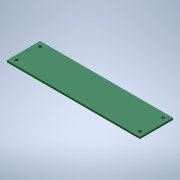
# Autodesk Inventor part: tapa
Saved by Autodesk Inventor 2021 (Build 250183000, 183)
## iProperties
Created: 2021-03-08
Part Number: tapa
Material: Steel, Mild, Welded
Document SubType Name: Modeling
Designer: Usuario
Density: 7.85 g/cm^3
Appearance: Smooth - Dark Sea Green
Author: Usuario
Autodesk Inventor part; units mm, degrees
ref_plane "YZ Plane" through (0, 0, 0) normal (1, 0, 0) x (0, 1, 0)
ref_plane "XZ Plane" through (0, 0, 0) normal (0, 1, 0) x (-1, 0, 0)
ref_plane "XY Plane" through (0, 0, 0) normal (0, 0, 1) x (1, 0, 0)
sketch "Sketch1" plane through (0, 0, 0) normal (0, 1, 0) x (-1, 0, 0)
  line L0 (76, 19) -> (-76, 19)
  line L1 (-76, 19) -> (-76, -19)
  line L2 (-76, -19) -> (76, -19)
  line L3 (76, -19) -> (76, 19)
  line L4 (76, 19) -> (-76, -19) construction
  line L5 (-76, 19) -> (76, -19) construction
  point P0 (0, 0)
  dimension "d0" = 152
  dimension "d1" = 38
  constraints: 12 end point, 2 midpoint, 2 parallel, 1 horizontal, 1 perpendicular
  measures "d0" distance of L2.end L1.end
  measures "d1" distance of L1.end L0.end
extrude "Extrusion1" add sketch "Sketch1" along normal blind 2
sketch "Sketch2" plane through (0, 0, 0) normal (0, -1, 0) x (1, 0, 0)
  line L0 (76, 19) -> (76, -19) projected
  line L1 (-76, 19) -> (76, 19) projected
  line L2 (-76, -19) -> (-76, 19) projected
  line L3 (76, -19) -> (-76, -19) projected
  line L4 (-76, -19) -> (-76, 19) projected
  line L5 (-76, 19) -> (76, 19) projected
  line L6 (-76, -19) -> (76, -19)
  line L7 (76, -19) -> (76, 19)
  line L8 (76, 19) -> (-76, 19)
  line L9 (-76, 19) -> (-76, -19)
  line L10 (-76, -19) -> (-75.15, -19)
  line L11 (76, -19) -> (-76, -19) projected
  line L12 (76, 19) -> (76, 18.15)
  line L13 (76, 19) -> (76, -19) projected
  line L14 (-75.15, -18.15) -> (75.15, -18.15)
  line L15 (75.15, -18.15) -> (75.15, 18.15)
  line L16 (75.15, 18.15) -> (-75.15, 18.15)
  line L17 (-75.15, 18.15) -> (-75.15, -18.15)
  line L18 (75.15, -18.15) -> (74.4, -18.15)
  line L19 (-75.15, 18.15) -> (-74.4, 18.15)
  line L20 (74.4, -17.4) -> (-74.4, -17.4)
  line L21 (-74.4, -17.4) -> (-74.4, 17.4)
  line L22 (-74.4, 17.4) -> (74.4, 17.4)
  line L23 (74.4, 17.4) -> (74.4, -17.4)
  point P0 (0, 0)
  constraints: 32 end point, 6 parallel, 4 point on line, 3 horizontal, 3 perpendicular
extrude "Extrusion2" cut sketch "Sketch2" against normal blind 0.75 contours L17 L16 L15 L14
sketch "Sketch3" plane through (0, 0, 0) normal (0, -1, 0) x (1, 0, 0)
  line L0 (-75.15, 18.15) -> (75.15, 18.15) projected
  line L1 (-75.15, -18.15) -> (-75.15, 18.15) projected
  line L2 (75.15, -18.15) -> (-75.15, -18.15) projected
  line L3 (75.15, 18.15) -> (75.15, -18.15) projected
  line L4 (-74.4, -17.4) -> (74.4, -17.4) projected
  line L5 (-74.4, 17.4) -> (-74.4, -17.4) projected
  line L6 (74.4, 17.4) -> (-74.4, 17.4) projected
  line L7 (74.4, -17.4) -> (74.4, 17.4) projected
  line L8 (76, 19) -> (76, -19) projected
  line L9 (-76, 19) -> (76, 19) projected
  line L10 (-76, -19) -> (-76, 19) projected
  line L11 (76, -19) -> (-76, -19) projected
  line L12 (-75.15, -18.15) -> (-75.15, 18.15) projected
  line L13 (-75.15, 18.15) -> (75.15, 18.15) projected
  line L14 (75.15, 18.15) -> (75.15, -18.15) projected
  line L15 (75.15, -18.15) -> (-75.15, -18.15) projected
  line L16 (-74.4, 17.4) -> (-74.4, -17.4) projected
  line L17 (-74.4, -17.4) -> (74.4, -17.4) projected
  line L18 (74.4, -17.4) -> (74.4, 17.4) projected
  line L19 (74.4, 17.4) -> (-74.4, 17.4) projected
  line L20 (-74.4, 17.4) -> (-74.4, -17.4) projected
  line L21 (-74.4, 17.4) -> (-66.4, 17.4)
  line L22 (-66.4, 17.4) -> (-66.4, 9.4)
  line L23 (-66.4, 9.4) -> (-74.4, 9.4)
  line L24 (-74.4, 9.4) -> (-74.4, 17.4)
  line L25 (-74.4, -17.4) -> (-66.4, -17.4)
  line L26 (-66.4, -17.4) -> (-66.4, -9.4)
  line L27 (-66.4, -9.4) -> (-74.4, -9.4)
  line L28 (-74.4, -9.4) -> (-74.4, -17.4)
  line L29 (74.4, -17.4) -> (74.4, 17.4) projected
  line L30 (74.4, 17.4) -> (66.4, 17.4)
  line L31 (66.4, 17.4) -> (66.4, 9.4)
  line L32 (66.4, 9.4) -> (74.4, 9.4)
  line L33 (74.4, 9.4) -> (74.4, 17.4)
  line L34 (-74.4, -17.4) -> (74.4, -17.4) projected
  line L35 (74.4, -17.4) -> (66.4, -17.4)
  line L36 (66.4, -17.4) -> (66.4, -9.4)
  line L37 (66.4, -9.4) -> (74.4, -9.4)
  line L38 (74.4, -9.4) -> (74.4, -17.4)
  line L39 (-74.4, -17.4) -> (-66.4, -9.4)
  line L40 (-66.4, -17.4) -> (-74.4, -9.4)
  line L41 (-74.4, 9.4) -> (-66.4, 17.4)
  line L42 (74.4, 17.4) -> (-74.4, 17.4) projected
  line L43 (-66.4, 9.4) -> (-74.4, 17.4)
  circle A0 centre (-70.4, -13.4) radius 1.65
  circle A1 centre (-70.4, 13.4) radius 1.65
  line L44 (66.4, -17.4) -> (74.4, -9.4)
  line L45 (66.4, 9.4) -> (74.4, 17.4)
  line L46 (74.4, 9.4) -> (66.4, 17.4)
  line L47 (74.4, -17.4) -> (66.4, -9.4)
  circle A2 centre (70.4, -13.4) radius 1.65
  circle A3 centre (70.4, 13.4) radius 1.65
  point P0 (0, 0)
  dimension "d14" = 8
  dimension "d15" = 8
  dimension "d16" = 8
  dimension "d17" = 8
  dimension "d18" = 8
  dimension "d19" = 8
  dimension "d20" = 8
  dimension "d21" = 8
  dimension "d22" = 3.3
  dimension "d23" = 3.3
  dimension "d24" = 3.3
  dimension "d25" = 3.3
  constraints: 48 end point, 8 parallel, 4 centre point, 4 horizontal, 4 midpoint, 4 perpendicular
  measures "d14" distance of L22.end L23.end
  measures "d15" distance of L21.end L22.end
  measures "d16" distance of L27.end L26.end
  measures "d17" distance of L26.end L25.end
  measures "d18" distance of L32.end L31.end
  measures "d19" distance of L31.end L30.end
  measures "d20" distance of L36.end L37.end
  measures "d21" distance of L35.end L36.end
  measures "d22" diameter of A0
  measures "d23" diameter of A1
  measures "d24" diameter of A2
  measures "d25" diameter of A3
extrude "Extrusion3" cut sketch "Sketch3" against normal blind 3 contours A0 L40 L39 | L39 L40 A0 | L40 L39 A0 | A0 L39 L40 | A2 L47 L44 | L44 L47 A2 | A1 L43 L41 | L41 L43 A1 | L47 L44 A2 | A2 L44 L47 | A1 L41 L43 | L43 L41 A1 | A3 L45 L46 | L46 L45 A3 | A3 L45 L46 | L46 L45 A3
body "Solid1"
